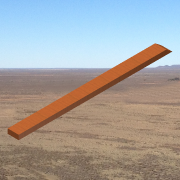
# Autodesk Inventor part: pole_EdgeRimHoriz
Saved by Autodesk Inventor 2013 SP2 (Build 170200200, 200)
## iProperties
Created: 2013-09-03
Part Number: pole_EdgeRimHoriz
Material: Wood (Cherry)
Document SubType Name: Modeling
Designer: Dave
Mass: 2323.84 g
Surface Area: 3574.83 cm^2
Volume: 4647.68 cm^3
Density: 0.5 g/cm^3
Author: Dave
Autodesk Inventor part; units mm, degrees
ref_plane "YZ Plane" through (0, 0, 0) normal (1, 0, 0) x (0, 1, 0)
ref_plane "XZ Plane" through (0, 0, 0) normal (0, 1, 0) x (-1, 0, 0)
ref_plane "XY Plane" through (0, 0, 0) normal (0, 0, 1) x (1, 0, 0)
sketch "Sketch1" plane through (0, 0, 0) normal (1, 0, 0) x (0, 1, 0)
  line L0 (0, 0) -> (38.1, 0)
  line L1 (38.1, 0) -> (38.1, -1189.8671)
  line L2 (38.1, -1239.52) -> (0, -1239.52) construction
  line L3 (0, -1239.52) -> (0, 0)
  line L4 (0, -1239.52) -> (38.1, -1189.8671)
  line L5 (0, -1239.52) -> (104.052, -1239.52) construction
  dimension "d0" = 38.1
  dimension "d1" = 1239.52
  dimension "d3" = 37.5
  constraints: 12 end point, 2 horizontal, 2 parallel, 1 perpendicular
  measures "d0" distance of L0.start L0.end
  measures "d1" distance of L2.end L0.start
  measures "d3" angle of L4 L3
extrude "Extrusion1" add sketch "Sketch1" along normal blind 88.9
sketch "Sketch2" plane through (0, 38.1, -1189.8671) normal (0, 0.7933533, -0.6087614) x (1, 0, 0)
  line L0 (0, 0) -> (88.9, 0) projected
  line L1 (88.9, 62.5861) -> (88.9, 0) projected
  circle A0 centre (63.5, 31.293) radius 5.3496
  circle A1 centre (25.4, 31.293) radius 5.3496
  point P0 (0, -920.7912)
  dimension "d6" = 25.4
  dimension "d9" = 38.1
  constraints: 2 centre point, 1 horizontal, 2 other
  measures "d6" distance from line of L1 A0.centre
  measures "d9" distance of A0.centre A1.centre
hole "Hole1" at (25.4, 19.05, -1214.6936) at (63.5, 19.05, -1214.6936) direction (0, -0.7933533, 0.6087614) diameter 6.35 depth 25.4 tip angle 118
body "Solid1"
